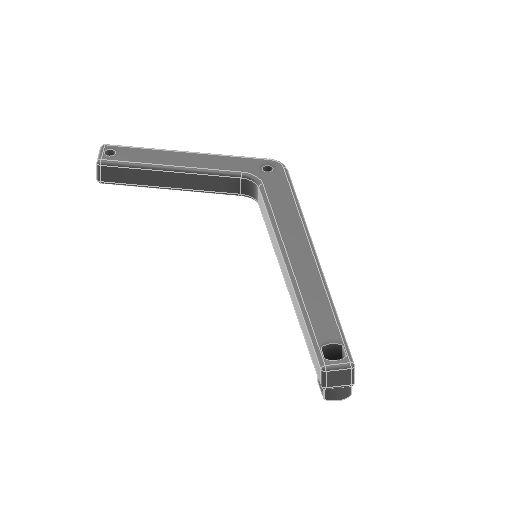
# Autodesk Inventor part: rocker
Saved by Autodesk Inventor 2025 (Build 290162010, 162A)
## iProperties
Created: 2024-08-06
Part Number: rocker
Material: PVC, Unplasticized
Document SubType Name: Modeling
Designer: Pauline Simonnet
Density: 1.29 g/cm^3
Appearance: Smooth - Black
Author: Pauline Simonnet
Autodesk Inventor part; units mm, degrees
ref_plane "YZ Plane" through (0, 0, 0) normal (1, 0, 0) x (0, 1, 0)
ref_plane "XZ Plane" through (0, 0, 0) normal (0, 1, 0) x (-1, 0, 0)
ref_plane "XY Plane" through (0, 0, 0) normal (0, 0, 1) x (1, 0, 0)
sketch "Sketch1" plane through (0, 0, 0) normal (0, 1, 0) x (-1, 0, 0)
  line L0 (-501.243392, -114.459807) -> (-592.595257, -181.302527)
  line L1 (-592.595257, -181.302527) -> (-790.515805, -48.772064)
  line L2 (-803.86928, -68.714098) -> (-591.985169, -210.594764)
  line L3 (-790.515805, -48.772064) -> (-803.86928, -68.714098)
  line L4 (-501.243392, -114.459807) -> (-487.071167, -133.828546)
  line L5 (-487.071167, -133.828546) -> (-591.985169, -210.594764)
  circle A0 centre (-592.348209, -193.164076) radius 4
  circle A1 centre (-500.613526, -128.868251) radius 4
  line L6 (-591.985169, -210.594764) -> (-578.40438, -190.31326) construction
  line L7 (-591.985169, -210.594764) -> (-603.360476, -195.048485) construction
  line L8 (-780.974109, -78.930211) -> (-792.122045, -71.465392)
  line L9 (-772.34999, -66.050981) -> (-783.497926, -58.586162)
  line L10 (-777.923958, -62.318572) -> (-786.548077, -75.197802) construction
  line L11 (-797.192543, -58.743081) -> (-765.20293, -80.163788) construction
  arc A2 (-780.974109, -78.930211) -> (-772.34999, -66.050981) centre (-782.236017, -68.758187) ccw
  arc A3 (-783.497926, -58.586162) -> (-792.122045, -71.465392) centre (-782.236017, -68.758187) ccw
  point P0 (0, 0)
  point P1 (-782.236017, -68.758187)
  dimension "d17" = 110
  dimension "d19" = 24
  dimension "d21" = 24
  dimension "d22" = 245
  dimension "d23" = 90
  dimension "d24" = 10
  dimension "d25" = 8
  dimension "d26" = 90
  dimension "d27" = 10
  dimension "d28" = 8
  dimension "d29" = 12
  dimension "d30" = 8
  dimension "d37" = 120
  dimension "d47" = 15.5
  dimension "d48" = 4.25
  dimension "d49" = 18
  dimension "d50" = 10.25
  constraints: 24 end point, 5 midpoint, 4 centre point, 4 point on circle, 2 perpendicular, 1 point on line
  measures "d17" angle of L1 L0
  measures "d19" distance between parallel lines of L1 L2
  measures "d21" distance between parallel lines of L0 L5
  measures "d22" distance from line of L3 A0.centre
  measures "d23" angle of L2 L6
  measures "d24" distance from line of A0.centre L6
  measures "d25" diameter of A0
  measures "d26" angle of L7 L5
  measures "d27" distance from line of A0.centre L7
  measures "d28" diameter of A1
  measures "d29" distance from line of L5 A1.centre
  measures "d30" distance from line of A1.centre L4
  measures "d37" distance from line of A0.centre L4
  measures "d47" distance between parallel lines of L9 L8
  measures "d48" distance between parallel lines of L8 L2
  measures "d49" distance from line of L3 point (-782.236, -68.758)
  measures "d50" radius of A2
extrude "Extrusion1" add sketch "Sketch1" along normal blind 20
fillet "Fillet1" radius 15 1 edges at (592.5953, 10, -181.3025)
fillet "Fillet2" radius 3 3 edges at (592.6642, 20, -177.9916) (542.6812, 20, -144.7801) (695.9191, 20, -112.1154)
fillet "Fillet3" radius 15 1 edges at (591.9852, 10, -210.5948)
fillet "Fillet4" radius 3 3 edges at (592.0541, 20, -207.2839) (702.2908, 20, -136.7325) (535.29, 20, -169.1106)
fillet "Fillet5" radius 3 3 edges at (592.0541, 0, -207.2839) (702.2908, 0, -136.7325) (535.29, 0, -169.1106)
fillet "Fillet6" radius 3 3 edges at (592.6642, 0, -177.9916) (542.6812, 0, -144.7801) (695.9191, 0, -112.1154)
fillet "Fillet7" radius 3 8 edges at (500.7245, 19.1213, -115.1689) (501.2434, 10, -114.4598) (500.7245, 0.8787, -115.1689) (494.1573, 0, -124.1442) (487.59, 0.8787, -133.1194) (487.0712, 10, -133.8285) (487.59, 19.1213, -133.1194) (494.1573, 20, -124.1442)
fillet "Fillet8" radius 3 8 edges at (803.3804, 19.1213, -67.984) (803.8693, 10, -68.7141) (803.3804, 0.8787, -67.984) (797.1925, 0, -58.7431) (791.0047, 0.8787, -49.5022) (790.5158, 10, -48.7721) (791.0047, 19.1213, -49.5022) (797.1925, 20, -58.7431)
sketch "Sketch5" plane through (0, 0, 0) normal (0, -1, 0) x (1, 0, 0)
  arc A0 (792.122045, -71.465392) -> (783.497926, -58.586162) centre (782.236017, -68.758187) ccw
  line L0 (789.692235, -52.934002) -> (602.991668, -177.951404)
  line L1 (786.408605, -55.132769) -> (768.048323, -67.427079)
  line L2 (794.22811, -71.258628) -> (779.980833, -80.798811)
  line L3 (795.989788, -72.48596) -> (780.444734, -82.895153)
  line L4 (780.974109, -78.930211) -> (792.122045, -71.465392)
  arc A1 (795.989788, -72.48596) -> (786.408605, -55.132769) centre (782.236017, -68.758187) ccw
  arc A2 (768.048323, -67.427079) -> (780.444734, -82.895153) centre (782.236017, -68.758187) ccw
  arc A3 (794.22811, -71.258628) -> (784.133713, -56.656069) centre (782.236017, -68.758187) ccw
  arc A4 (770.323215, -65.903779) -> (779.980833, -80.798811) centre (782.236017, -68.758187) ccw
  point P0 (0, 0)
  point P1 (784.133713, -56.656069)
  dimension "d69" = 0
  dimension "d70" = 0
  dimension "d73" = 1
  dimension "d74" = 2
  dimension "d75" = 2
  dimension "d76" = 2
  dimension "d77" = 2
  constraints: 8 point on circle, 6 end point, 4 centre point, 4 point on line, 3 parallel, 1 coincident
  measures "d69" distance of A0.centre A3.centre
  measures "d70" distance of A0.centre A3.centre
  measures "d73" distance between parallel lines of L4 L2
  measures "d74" distance between parallel lines of L2 L3
  measures "d75" radial gap between concentric circles of A4 A2
  measures "d76" radial gap between concentric circles of A3 A1
  measures "d77" radial gap between concentric circles of A0 A3
extrude "Extrusion4" add sketch "Sketch5" along normal blind 10 contours A1 L3 A2 L0 A4 L2 A3
sketch "Sketch6" plane through (0, -10, 0) normal (0, -1, 0) x (1, 0, 0)
  arc A0 (795.989788, -72.48596) -> (796.423711, -70.089294) centre (782.236017, -68.758187) ccw
  arc A1 (778.063429, -82.383605) -> (780.444734, -82.895153) centre (782.236017, -68.758187) ccw
  line L0 (795.989788, -72.48596) -> (780.444734, -82.895153)
  line L1 (786.408605, -55.132769) -> (789.692235, -52.934002)
  line L2 (786.408605, -55.132769) -> (768.048323, -67.427079)
  arc A2 (795.989788, -72.48596) -> (786.408605, -55.132769) centre (782.236017, -68.758187) ccw
  arc A3 (768.048323, -67.427079) -> (780.444734, -82.895153) centre (782.236017, -68.758187) ccw
  point P0 (0, 0)
  constraints: 4 end point, 4 point on circle, 2 centre point, 1 coincident, 1 collinear
extrude "Extrusion5" add sketch "Sketch6" along normal blind 2
fillet "Fillet10" radius 2 1 edges at (788.2173, 0, -77.6906)
body "Solid1"
